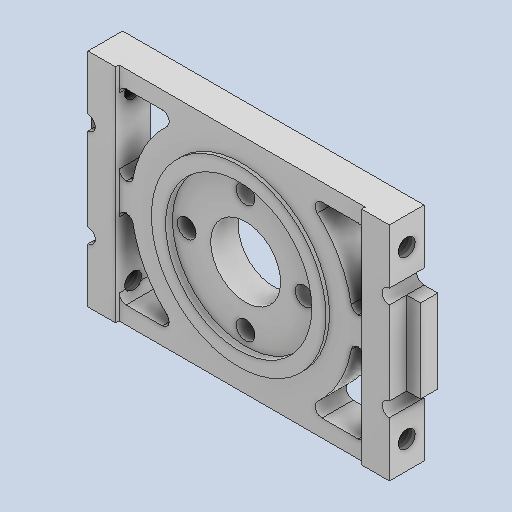
# Autodesk Inventor part: Shoulder_horn_frame
Saved by Autodesk Inventor 2022.4 (Build 264492000, 492)
## iProperties
Created: 2021-09-24
Part Number: Shoulder_horn_frame
Material: アルミニウム 2014-T4
Document SubType Name: Modeling
Designer: Masato Kubotera
Density: 2.8 g/cm^3
Appearance: 滑らか - 淡い灰色
Mass: 14.1002 g
Surface Area: 41.1044 cm^2
Volume: 5.03579 cm^3
Description: A2017 T5
Author: Masato Kubotera
Autodesk Inventor part; units mm, degrees
ref_plane "YZ Plane" through (0, 0, 0) normal (1, 0, 0) x (0, 1, 0)
ref_plane "XZ Plane" through (0, 0, 0) normal (0, 1, 0) x (-1, 0, 0)
ref_plane "XY Plane" through (0, 0, 0) normal (0, 0, 1) x (1, 0, 0)
sketch "スケッチ1" plane through (0, 0, 0) normal (0, 0, 1) x (1, 0, 0)
  line L0 (-21.75, 16) -> (21.75, 16)
  line L1 (21.75, -16) -> (-21.75, -16)
  line L2 (-21.75, 16) -> (21.75, -16) construction
  line L3 (21.75, 16) -> (-21.75, -16) construction
  circle A0 centre (0, 0) radius 10.5 construction
  line L4 (0, 16) -> (0, -16) construction
  circle A1 centre (0, 8.5) radius 1.35
  circle A2 centre (-8.5, 0) radius 1.35
  circle A3 centre (0, -8.5) radius 1.35
  circle A4 centre (8.5, 0) radius 1.35
  line L5 (-21.75, 6) -> (-23.75, 6)
  line L6 (-23.75, 6) -> (-23.75, -6)
  arc A5 (-21.75, 6) -> (-21.75, 8.1) centre (-21.75, 7.05) ccw
  line L7 (-21.75, 8.1) -> (-21.75, 16)
  line L8 (-23.75, 0) -> (23.75, 0) construction
  line L9 (-21.75, -6) -> (-23.75, -6)
  arc A6 (-21.75, -8.1) -> (-21.75, -6) centre (-21.75, -7.05) ccw
  line L10 (-21.75, -8.1) -> (-21.75, -16)
  line L11 (23.75, 6) -> (23.75, -6)
  arc A7 (21.75, 8.1) -> (21.75, 6) centre (21.75, 7.05) ccw
  line L12 (21.75, 8.1) -> (21.75, 16)
  line L13 (21.75, -6) -> (23.75, -6)
  line L14 (21.75, -8.1) -> (21.75, -16)
  arc A8 (21.75, -6) -> (21.75, -8.1) centre (21.75, -7.05) ccw
  line L15 (21.75, 6) -> (23.75, 6)
  line L16 (-21.75, 13.55) -> (-15.75, 13.55) construction
  line L17 (-15.75, 13.55) -> (-15.75, 10.45) construction
  line L18 (-15.75, 10.45) -> (-21.75, 10.45) construction
  line L19 (-15.75, 12) -> (-21.75, 12) construction
  arc A9 (-8.587782, 13.5) -> (-15.874508, 2) centre (0, 0) ccw
  circle A10 centre (0, 0) radius 5.05
  line L20 (-15.874508, 2) -> (-17.75, 2)
  line L21 (-17.75, 2) -> (-17.75, 13.5)
  line L22 (-17.75, 13.5) -> (-8.587782, 13.5)
  circle A11 centre (0, 0) radius 10.55
  circle A12 centre (0, 0) radius 5 construction
  line L23 (-21.75, 6) -> (-21.75, -6)
  line L24 (21.75, 6) -> (21.75, -6)
  arc A13 (-15.874508, -2) -> (-8.587782, -13.5) centre (0, 0) ccw
  line L25 (-15.874508, -2) -> (-17.75, -2)
  line L26 (-17.75, -2) -> (-17.75, -13.5)
  line L27 (-17.75, -13.5) -> (-8.587782, -13.5)
  arc A14 (15.874508, 2) -> (8.587782, 13.5) centre (0, 0) ccw
  line L28 (17.75, 2) -> (17.75, 13.5)
  line L29 (17.75, 13.5) -> (8.587782, 13.5)
  line L30 (15.874508, -2) -> (17.75, -2)
  arc A15 (8.587782, -13.5) -> (15.874508, -2) centre (0, 0) ccw
  line L31 (17.75, -2) -> (17.75, -13.5)
  line L32 (17.75, -13.5) -> (8.587782, -13.5)
  line L33 (15.874508, 2) -> (17.75, 2)
  circle A16 centre (0, 0) radius 16.05
  circle A17 centre (0, 0) radius 12.6
  line L34 (-17.75, 13.5) -> (-17.75, 16)
  line L35 (17.75, 13.5) -> (17.75, 16)
  line L36 (-17.75, -13.5) -> (-17.75, -16)
  line L37 (17.75, -13.5) -> (17.75, -16)
  line L38 (17.75, -2) -> (17.75, 2)
  line L39 (-17.75, -2) -> (-17.75, 2.256219)
  point P0 (0, 0)
  point P1 (-6.538348, 13.5)
  point P2 (-8.680582, 13.5)
  point P3 (8.680582, 13.5)
  point P4 (15.924902, 2)
  point P5 (15.924902, -2)
  point P6 (8.680582, -13.5)
  point P7 (-8.680582, -13.5)
  point P8 (-15.924902, -2)
  point P9 (-15.924902, 2)
  point P10 (-1.265899, -16)
  point P11 (1.265899, -16)
  point P12 (1.265899, 16)
  point P13 (-1.265899, 16)
  dimension "d0" = 21
  dimension "d1" = 2.7
  dimension "d2" = 8.5
  dimension "d5" = 360
  dimension "d7" = 43.5
  dimension "d8" = 32
  dimension "d10" = 10
  dimension "d11" = 1.05
  dimension "d12" = 2
  dimension "d13" = 3.1
  dimension "d14" = 6
  dimension "d15" = 6
  dimension "d17" = 4
  dimension "d18" = 2.5
  dimension "d22" = 10
  dimension "d23" = 0.05
  dimension "d24" = 0.05
  dimension "d52" = 16
  dimension "d53" = 4
  dimension "d54" = 32.1
  dimension "d57" = 25.2
  constraints: 80 end point, 27 symmetric about line, 18 centre point, 17 point on circle, 10 point on line, 9 midpoint, 8 perpendicular, 7 coincident, 6 horizontal, 2 parallel, 2 vertical, 1 tangent, 15 other
  measures "d0" diameter of A0
  measures "d1" diameter of A1
  measures "d2" distance of point (0, 0) A1.centre
  measures "d7" distance of L0.end L0.start
  measures "d8" distance of L1.end L0.start
  measures "d10" distance of L0.start L5.start
  measures "d11" radius of A5
  measures "d12" distance of L5.start L5.end
  measures "d13" distance of L17.end L16.end
  measures "d14" distance of L16.start L16.end
  measures "d15" vertical distance of L5.end L19.end
  measures "d17" horizontal distance of L0.start L21.end
  measures "d18" vertical distance of L0.start L21.end
  measures "d22" diameter of A12
  measures "d23" radial gap between concentric circles of A12 A10
  measures "d24" radial gap between concentric circles of A11 A0
  measures "d52" radius of A9
  measures "d53" distance of L25.end L20.end
  measures "d54" diameter of A16
  measures "d57" diameter of A17
extrude "押し出し1" add sketch "スケッチ1" along normal blind 5 contours L0 L34 L21 L39 L26 L36 L1 L10 A6 L23 A5 L7 | L0 L12 A7 L24 A8 L14 L1 L37 L31 L38 L28 L35 | A17
extrude "押し出し2" add sketch "スケッチ1" along normal blind 4 contours A11
extrude "押し出し3" add sketch "スケッチ1" along normal blind 2.5 contours L23 L9 L6 L5 | L15 L11 L13 L24
sketch "スケッチ1 outline for 押し出し4" plane through (0, 0, 0) normal (0, 0, 1) x (1, 0, 0)
  arc A0 (-8.587782, 13.5) -> (-15.874508, 2) centre (0, 0) ccw
  line L0 (-15.874508, 2) -> (-17.75, 2)
  line L1 (-17.75, 2) -> (-17.75, -2)
  line L2 (-17.75, -2) -> (-15.874508, -2)
  arc A1 (-15.874508, -2) -> (-8.587782, -13.5) centre (0, 0) ccw
  line L3 (-8.587782, -13.5) -> (-17.75, -13.5)
  line L4 (-17.75, -13.5) -> (-17.75, -16)
  line L5 (-17.75, -16) -> (17.75, -16)
  line L6 (17.75, -16) -> (17.75, -13.5)
  line L7 (17.75, -13.5) -> (8.587782, -13.5)
  arc A2 (8.587782, -13.5) -> (15.874508, -2) centre (0, 0) ccw
  line L8 (15.874508, -2) -> (17.75, -2)
  line L9 (17.75, -2) -> (17.75, 2)
  line L10 (17.75, 2) -> (15.874508, 2)
  arc A3 (15.874508, 2) -> (8.587782, 13.5) centre (0, 0) ccw
  line L11 (8.587782, 13.5) -> (17.75, 13.5)
  line L12 (17.75, 13.5) -> (17.75, 16)
  line L13 (17.75, 16) -> (-17.75, 16)
  line L14 (-17.75, 16) -> (-17.75, 13.5)
  line L15 (-17.75, 13.5) -> (-8.587782, 13.5)
  circle A4 centre (0, 0) radius 10.55
extrude "押し出し4" add sketch "スケッチ1 outline for 押し出し4" along normal blind 4.5
fillet "フィレット1" radius 1 16 edges at (15.8745, 2, 2.25) (15.8745, -2, 2.25) (-15.8745, 2, 2.25) (-15.8745, -2, 2.25) (-8.5878, 13.5, 2.25) (8.5878, 13.5, 2.25) (8.5878, -13.5, 2.25) (-8.5878, -13.5, 2.25) (-17.75, 13.5, 2.25) (-17.75, -13.5, 2.25) (17.75, -13.5, 2.25) (17.75, 13.5, 2.25) (-17.75, -2, 2.25) (-17.75, 2, 2.25) (17.75, -2, 2.25) (17.75, 2, 2.25)
sketch "スケッチ2" plane through (-21.75, 8.1, 0) normal (-1, 0, 0) x (0, 0, 1)
  line L0 (0, 7.9) -> (0, 0) projected
  line L1 (0, -16.2) -> (0, -24.1) projected
  line L2 (2.5, -2.1) -> (5, -2.1) projected
  line L3 (2.5, -14.1) -> (5, -14.1) projected
  point P0 (0, -8.1)
  point P1 (2.5, 3.9)
  point P2 (2.5, -20.1)
  point P3 (0, -2.1)
  point P4 (0, -14.1)
  dimension "d30" = 2.5
  dimension "d32" = 2.5
  dimension "d50" = 6
  dimension "d51" = 6
  measures "d30" distance from line of L0 point (2.5, 3.9)
  measures "d32" distance from line of L1 point (2.5, -20.1)
  measures "d50" distance from line of point (2.5, 3.9) L2
  measures "d51" distance from line of point (2.5, -20.1) L3
hole "穴1" at (-21.75, 12, 2.5) at (-21.75, -12, 2.5) direction (1, 0, 0) diameter 2.459 depth 4 tip angle 118 thread size "M3x0.5" class "6H" standard "ISO Metric profile"
sketch "スケッチ3" plane through (21.75, 8.1, 0) normal (1, 0, 0) x (0, 0, -1)
  circle A0 centre (-2.5, 3.9) radius 1.2295 projected
  circle A1 centre (-2.5, -20.1) radius 1.2295 projected
  point P0 (0, -8.1)
  constraints: 2 coincident
hole "穴2" at (21.75, 12, 2.5) at (21.75, -12, 2.5) direction (-1, 0, 0) diameter 2.459 depth 4 tip angle 118 thread size "M3x0.5" class "6H" standard "ISO Metric profile"
equation "\"d24\" = d23"
equation "\"d32\" = d30"
equation "\"d50\" = d15"
equation "\"d51\" = d50"
